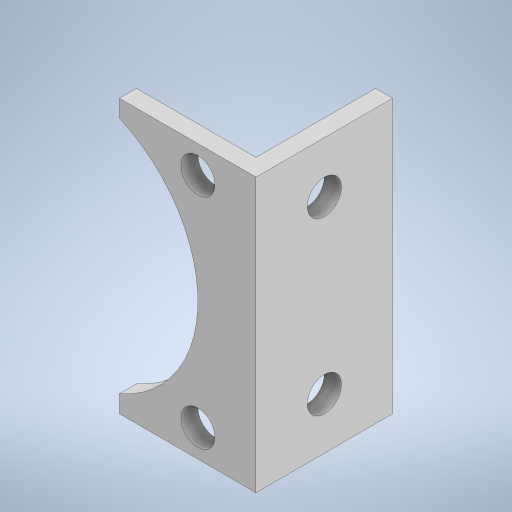
# Autodesk Inventor part: Frame Bracket
Saved by Autodesk Inventor 2023 (Build 270158000, 158)
## iProperties
Created: 2022-10-26
Part Number: Frame Bracket
Material: Generic
Document SubType Name: Modeling
Designer: tommy
Density: 1 g/cm^3
Appearance: Default
Author: tommy
Autodesk Inventor part; units mm, degrees
ref_plane "YZ Plane" through (0, 0, 0) normal (1, 0, 0) x (0, 1, 0)
ref_plane "XZ Plane" through (0, 0, 0) normal (0, 1, 0) x (-1, 0, 0)
ref_plane "XY Plane" through (0, 0, 0) normal (0, 0, 1) x (1, 0, 0)
sketch "Sketch1" plane through (0, 0, 0) normal (0, 1, 0) x (-1, 0, 0)
  line L0 (0, 0) -> (0, -25.4)
  line L1 (0, -25.4) -> (3.175, -25.4)
  line L2 (3.175, -25.4) -> (3.175, -3.175)
  line L3 (3.175, -3.175) -> (25.4, -3.175)
  line L4 (25.4, -3.175) -> (25.4, 0)
  line L5 (25.4, 0) -> (0, 0)
  dimension "d0" = 25.4
  dimension "d1" = 3.175
  dimension "d2" = 22.225
  dimension "d3" = 22.225
  constraints: 12 end point, 5 perpendicular, 1 vertical
  measures "d0" distance of L0.start L0.end
  measures "d1" distance of L0.end L1.end
  measures "d2" distance of L1.end L2.end
  measures "d3" distance of L2.end L3.end
extrude "Extrusion1" add sketch "Sketch1" along normal blind 50.8
sketch "Sketch2" plane through (-25.4, 0, 0) normal (0, 0, 1) x (1, 0, 0)
  line L0 (22.225, 0) -> (22.225, 50.8) projected
  line L1 (22.225, 0) -> (0, 0) projected
  line L2 (22.225, 50.8) -> (0, 50.8) projected
  circle A0 centre (14.605, 45.72) radius 3.175
  circle A1 centre (14.605, 5.08) radius 3.175
  circle A2 centre (-9.525, 25.4) radius 24.13
  line L3 (25.4, 0) -> (22.225, 0) projected
  dimension "d9" = 6.35
  dimension "d10" = 6.35
  constraints: 3 centre point
  measures "d9" diameter of A0
  measures "d10" diameter of A1
extrude "Extrusion2" cut sketch "Sketch2" against normal blind 63.5
sketch "Sketch3" plane through (0, 0, 0) normal (1, 0, 0) x (0, 0, -1)
  line L0 (25.4, 0) -> (25.4, 50.8) projected
  line L1 (0, 3.2295) -> (0, 47.5705) projected
  line L2 (0, 50.8) -> (25.4, 50.8) projected
  line L3 (25.4, 0) -> (3.175, 0) projected
  circle A0 centre (12.7, 9.525) radius 3.175
  circle A1 centre (12.7, 41.275) radius 3.175
  point P0 (0, 0)
  constraints: 2 centre point
extrude "Extrusion3" cut sketch "Sketch3" against normal blind 63.5
body "Solid1"
